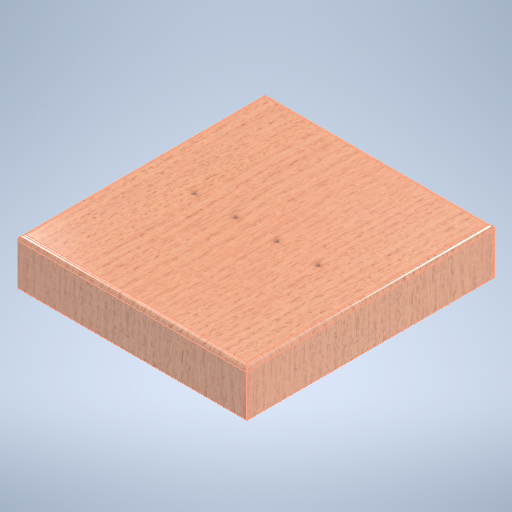
# Autodesk Inventor part: Block
Saved by Autodesk Inventor 2025.1 (Build 291241000, 241)
## iProperties
Created: 2024-09-17
Part Number: Block
Material: Wood (Cherry)
Document SubType Name: Modeling
Designer: ffogue
Density: 0.63 g/cm^3
Appearance: White Oak - Natural Medium Gloss
Author: ffogue
Autodesk Inventor part; units mm, degrees
ref_plane "YZ Plane" through (0, 0, 0) normal (1, 0, 0) x (0, 1, 0)
ref_plane "XZ Plane" through (0, 0, 0) normal (0, 1, 0) x (-1, 0, 0)
ref_plane "XY Plane" through (0, 0, 0) normal (0, 0, 1) x (1, 0, 0)
sketch "Sketch1" plane through (0, 0, 0) normal (0, 0, 1) x (1, 0, 0)
  line L0 (-125, -135) -> (125, -135)
  line L1 (125, -135) -> (125, 135)
  line L2 (125, 135) -> (-125, 135)
  line L3 (-125, 135) -> (-125, -135)
  line L4 (-125, -135) -> (125, 135) construction
  line L5 (125, -135) -> (-125, 135) construction
  point P0 (0, 0)
  dimension "d0" = 270
  dimension "d1" = 250
  constraints: 12 end point, 2 midpoint, 2 parallel, 1 horizontal, 1 perpendicular
  measures "d0" distance of L2.end L0.start
  measures "d1" distance of L0.start L0.end
extrude "Extrusion1" add sketch "Sketch1" along normal blind 50
fillet "Fillet1" radius 5 4 edges at (0, 135, 50) (125, 0, 50) (0, -135, 50) (-125, 0, 50)
sketch "Sketch2" plane through (0, 0, 50) normal (0, 0, 1) x (1, 0, 0)
  line L0 (125, 135) -> (-125, 135) projected
  line L1 (-125, 135) -> (-125, -135) projected
  point P0 (0, 0)
  point P1 (-67.5, 0)
  point P2 (-22.5, 0)
  point P3 (22.5, 0)
  point P4 (67.5, 0)
  point P5 (-125, 0)
  dimension "d5" = 135
  dimension "d6" = 45
  dimension "d7" = 45
  dimension "d8" = 45
  dimension "d10" = 67.5
  constraints: 3 horizontal alignment, 1 midpoint
  measures "d5" distance from line of L0 point (-67.5, 0)
  measures "d6" distance of point (-22.5, 0) point (-67.5, 0)
  measures "d7" distance of point (22.5, 0) point (-22.5, 0)
  measures "d8" distance of point (67.5, 0) point (22.5, 0)
  measures "d10" distance of point (-67.5, 0) point (0, 0)
hole "Hole1" at (-67.5, 0, 50) at (-22.5, 0, 50) at (22.5, 0, 50) at (67.5, 0, 50) direction (0, 0, -1) diameter 5 depth 50
equation "\"d7\" = d6"
equation "\"d8\" = d6"
body "Solid1"
